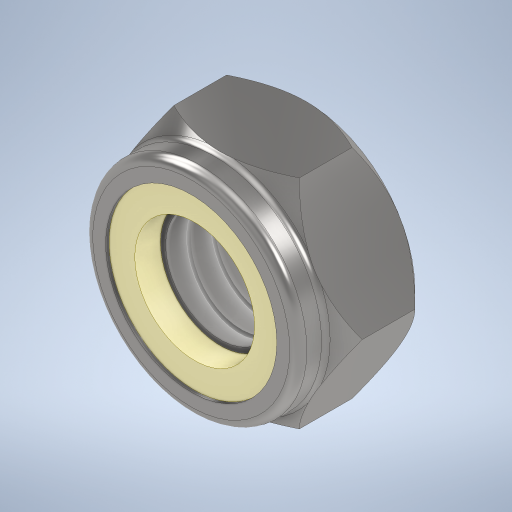
# Autodesk Inventor part: Gas Strut Locknut
Saved by Autodesk Inventor 2024 (Build 280153000, 153)
## iProperties
Created: 2024-09-05
Part Number: Gas Strut Locknut
Material: Stainless Steel
Document SubType Name: Modeling
Designer: Ishaan
Density: 8 g/cm^3
Appearance: Semi-Polished
Mass: 1.64294 g
Surface Area: 3.67732 cm^2
Volume: 0.205367 cm^3
Author: Ishaan
Autodesk Inventor part; units mm, degrees
ref_plane "YZ Plane" through (0, 0, 0) normal (1, 0, 0) x (0, 1, 0)
ref_plane "XZ Plane" through (0, 0, 0) normal (0, 1, 0) x (-1, 0, 0)
ref_plane "XY Plane" through (0, 0, 0) normal (0, 0, 1) x (1, 0, 0)
sketch "Sketch1" plane through (0, 0, 0) normal (0, 0, 1) x (1, 0, 0)
  circle A0 centre (0, 0) radius 7.332348
  line L0 (-3.666174, 6.35) -> (3.666174, 6.35)
  line L1 (3.666174, 6.35) -> (7.332348, 0)
  line L2 (7.332348, 0) -> (3.666174, -6.35)
  line L3 (3.666174, -6.35) -> (-3.666174, -6.35)
  line L4 (-3.666174, -6.35) -> (-7.332348, 0)
  line L5 (-7.332348, 0) -> (-3.666174, 6.35)
  point P0 (-7.332348, 0)
  point P1 (-7.332348, 0)
  point P2 (-3.666174, 6.35)
  point P3 (-3.666174, 6.35)
  point P4 (-3.666174, -6.35)
  point P5 (-3.666174, -6.35)
  point P6 (3.666174, -6.35)
  point P7 (3.666174, -6.35)
  point P8 (7.332348, 0)
  point P9 (7.332348, 0)
  dimension "d0" = 12.7
  constraints: 12 end point, 2 coincident, 1 horizontal, 16 other
  measures "d0" distance between parallel lines of L3 L0
extrude "Extrusion1" add sketch "Sketch1" along normal blind 5.08
chamfer "Chamfer1" distance 1 angle 45 2 edges at (-7.3323, 0, 0) (-7.3323, 0, 5.08)
extrude "Extrusion2" cut sketch "Sketch1" along normal through all contours L1 A0 | A0 L2 | L0 A0 | A0 L3 | L5 A0 | A0 L4
sketch "Sketch2" plane through (0, 0, 5.08) normal (0, 0, 1) x (1, 0, 0)
  circle A0 centre (0, 0) radius 6.332348
  circle A1 centre (0, 0) radius 6.25
  point P0 (2.236519, -6.35)
  point P1 (6.617521, 1.238118)
  dimension "d9" = 12.5
  constraints: 1 centre point, 1 coincident, 1 other
  measures "d9" diameter of A1
extrude "Extrusion3" add sketch "Sketch2" along normal blind 1.651 contours A1
fillet "Fillet1" radius 0.5 3 edges at (-6.25, 0, 5.08) (-6.3323, 0, 5.08) (-6.25, 0, 6.731)
sketch "Sketch3" plane through (0, 0, 6.731) normal (0, 0, 1) x (1, 0, 0)
  circle A0 centre (0, 0) radius 5
  dimension "d13" = 10
  constraints: 1 centre point, 1 coincident
  measures "d13" diameter of A0
extrude "Extrusion4" cut sketch "Sketch3" against normal blind 1.7
sketch "Sketch4" plane through (0, 0, 5.031) normal (0, 0, 1) x (1, 0, 0)
  circle A0 centre (0, 0) radius 5 projected
extrude "Extrusion5" add sketch "Sketch4" along normal blind 1.5 separate body
sketch "Sketch5" plane through (0, 0, 6.531) normal (0, 0, 1) x (1, 0, 0)
  circle A0 centre (0, 0) radius 5 projected
  constraints: 1 coincident
hole "Hole1" at (0, 0, 6.531) direction (0, 0, -1) diameter 6.4008 end through all bodies 1 thread size "5/16-18 UNC" class "2B" standard "ANSI Unified Screw Threads"
sketch "Sketch6" plane through (0, 0, 5.031) normal (0, 0, -1) x (-1, 0, 0)
  circle A0 centre (0, 0) radius 3.2004 projected
  constraints: 1 coincident
hole "Hole2" at (0, 0, 5.031) direction (0, 0, 1) diameter 7 end through all bodies 2
chamfer "Chamfer2" distance 0.25 angle 45 1 edges at (0, 3.2004, 0)
body "Solid1"
